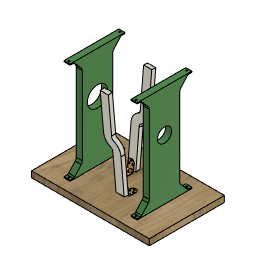
Ventilator_Mk_1_v11 (Autodesk Fusion 360 design; units mm, degrees)
Autodesk Fusion 360 part; units mm, degrees
sketch "Base" plane through (0, 0, 0) normal (0, 0, 1) x (1, 0, 0)
  line L0 (-114.3, 47.625) -> (114.3, 47.625)
  line L1 (114.3, 47.625) -> (114.3, -47.625)
  line L2 (114.3, -47.625) -> (-114.3, -47.625)
  line L3 (-114.3, -47.625) -> (-114.3, 47.625)
  line L4 (-114.3, 47.625) -> (114.3, -47.625) construction
  line L5 (114.3, 47.625) -> (-114.3, -47.625) construction
  line L6 (-95.25, 47.625) -> (-95.25, -47.625)
  line L7 (95.25, 47.625) -> (95.25, -47.625)
  line L8 (-38.1, 47.625) -> (-38.1, -47.625)
  line L9 (38.1, 47.625) -> (38.1, -47.625)
  line L10 (184.15, -117.475) -> (-184.15, -117.475)
  line L11 (-184.15, -117.475) -> (-184.15, 117.475)
  line L12 (-184.15, 117.475) -> (184.15, 117.475)
  line L13 (184.15, 117.475) -> (184.15, -117.475)
  line L14 (38.1323, 0.889) -> (15.9073, 0.889)
  line L15 (19.05, -15.9073) -> (19.05, -38.1323)
  circle A0 centre (22.86, -22.2573) radius 2.54
  circle A1 centre (34.29, -22.2573) radius 2.54
  line L16 (-114.3, -47.625) -> (-114.3, 47.625)
  line L17 (114.3, 47.625) -> (114.3, -47.625)
  line L18 (-114.3, 47.625) -> (-95.25, 47.625)
  line L19 (-95.25, 47.625) -> (-95.25, 85.725)
  line L20 (-95.25, 85.725) -> (-114.3, 85.725)
  line L21 (-114.3, 85.725) -> (-114.3, 47.625)
  line L22 (-114.3, -47.625) -> (-95.25, -47.625)
  line L23 (-95.25, -47.625) -> (-95.25, -85.725)
  line L24 (-95.25, -85.725) -> (-114.3, -85.725)
  line L25 (-114.3, -85.725) -> (-114.3, -47.625)
  line L26 (114.3, 47.625) -> (95.25, 47.625)
  line L27 (95.25, 47.625) -> (95.25, 85.725)
  line L28 (95.25, 85.725) -> (114.3, 85.725)
  line L29 (114.3, 85.725) -> (114.3, 47.625)
  line L30 (114.3, -47.625) -> (95.25, -47.625)
  line L31 (95.25, -47.625) -> (95.25, -85.725)
  line L32 (95.25, -85.725) -> (114.3, -85.725)
  line L33 (114.3, -85.725) -> (114.3, -47.625)
  line L34 (-95.25, -73.025) -> (-114.3, -73.025)
  line L35 (-114.3, 73.025) -> (-95.25, 73.025)
  line L36 (95.25, 73.025) -> (114.3, 73.025)
  line L37 (95.25, -73.025) -> (114.3, -73.025)
  line L38 (-95.25, -73.025) -> (-114.3, -85.725) construction
  line L39 (-114.3, 73.025) -> (-95.25, 85.725) construction
  line L40 (95.25, 73.025) -> (114.3, 85.725) construction
  line L41 (95.25, -85.725) -> (114.3, -73.025) construction
  point P0 (34.29, -22.2573)
  point P1 (22.86, -22.2573)
  point P2 (38.1, -4.445)
  point P3 (-38.1, 4.445)
  point P4 (38.1, -10.795)
  point P5 (-38.1, 10.795)
  point P6 (-104.775, -79.375)
  point P7 (-104.775, 79.375)
  point P8 (104.775, 79.375)
  point P9 (104.775, -79.375)
  dimension "d1" = 95.25
  dimension "d2" = 228.6
  dimension "d3" = 19.05
  dimension "d4" = 19.05
  dimension "d7" = 76.2
  dimension "d8" = 76.2
  dimension "d13" = -69.85
  dimension "d103" = 43.18
  dimension "d104" = 43.18
  dimension "d105" = 6.35
  dimension "d106" = 6.35
  dimension "d216" = 38.1
  dimension "d217" = 38.1
  dimension "d218" = 38.1
  dimension "d219" = 38.1
  dimension "d220" = 12.7
  dimension "d221" = 12.7
  constraint horizontal L0
  constraint perpendicular L0 L1
  constraint parallel L0 L2
  constraint parallel L1 L3
  constraint coincident L4 origin
  constraint coincident L5 origin
  constraint coincident L0 L6.start
  constraint coincident L2 L6.end
  constraint parallel L3 L6
  constraint coincident L0 L7.start
  constraint coincident L2 L7.end
  constraint parallel L6 L7
  constraint coincident L0 L8.start
  constraint coincident L2 L8.end
  constraint perpendicular L2 L8
  constraint coincident L0 L9.start
  constraint coincident L2 L9.end
  constraint perpendicular L2 L9
  constraint coincident L9 P2
  constraint coincident L8 P3
  constraint coincident L9 P4
  constraint coincident L8 P5
  constraint vertical L16
  constraint vertical L17
  constraint horizontal L18
  constraint vertical L19
  constraint horizontal L20
  constraint vertical L21
  constraint collinear L6 L19
  constraint horizontal L22
  constraint vertical L23
  constraint horizontal L24
  constraint vertical L25
  constraint collinear L6 L23
  constraint collinear L2 L22
  constraint horizontal L26
  constraint vertical L27
  constraint horizontal L28
  constraint vertical L29
  constraint collinear L7 L27
  constraint horizontal L30
  constraint vertical L31
  constraint horizontal L32
  constraint vertical L33
  constraint collinear L7 L31
  constraint coincident L23 L34.start
  constraint coincident L25 L34.end
  constraint perpendicular L25 L34
  constraint coincident L19 L35.end
  constraint perpendicular L19 L35
  constraint coincident L27 L36.start
  constraint coincident L29 L36.end
  constraint perpendicular L29 L36
  constraint coincident L31 L37.start
  constraint coincident L33 L37.end
  constraint perpendicular L33 L37
  constraint horizontal L34.end L37.start
  constraint horizontal L35.start L36.start
  constraint midpoint P6 L38
  constraint parallel L40 L41
  constraint midpoint L39 P7
  constraint midpoint L40 P8
  constraint midpoint L41 P9
  measures "d1" distance of L0.end L1.end
  measures "d2" distance of L1 L3
  measures "d3" distance of L3 L6
  measures "d4" distance of L1 L7
  measures "d7" distance of L3 L8
  measures "d8" distance of L1 L9
  measures "d47" distance of P1
  measures "d48" distance of P0
  measures "d49" distance of P0
  measures "d103" distance of L9.end P2
  measures "d104" distance of L8.start P3
  measures "d105" distance of P2 P4
  measures "d106" distance of P3 P5
  measures "d216" distance of L22 L24
  measures "d217" distance of L18 L20
  measures "d218" distance of L26 L28
  measures "d219" distance of L30 L32
  measures "d220" distance of L24 L34
  measures "d221" distance of L20 L35
extrude "Stand Extrude" add sketch "Base" along normal blind 317.5 contours L0 L2 L3 L6 L16 L18 L22 | L0 L1 L2 L7 L17 L26 L30 makes body 1 at (-95.25, 15.875, 105.8333) makes body 2 at (114.3, 15.875, 105.8333)
extrude "StandBaseExtrude" add sketch "Base" along normal blind 31.75 contours L0 L18 L19 L21 L35 | L2 L22 L23 L25 L34 | L0 L26 L27 L29 L36 | L2 L30 L31 L33 L37 bodies 1 2
extrude "StandBaseMountExtrude" add sketch "Base" along normal blind 3.175 contours L19 L20 L21 L35 | L23 L24 L25 L34 | L27 L28 L29 L36 | L31 L32 L33 L37 bodies 1 2
extrude "BaseExtrude" add sketch "Base" against normal blind 19.05 separate body contours L0 L18 L19 L21 L35 | L0 L2 L3 L6 L16 L18 L22 | L0 L2 L6 L8 | L2 L22 L23 L25 L34 | L19 L20 L21 L35 | L0 L2 L8 L9 | L23 L24 L25 L34 | L0 L2 L7 L9 | L0 L26 L27 L29 L36 | L0 L1 L2 L7 L17 L26 L30 | L2 L30 L31 L33 L37 | L27 L28 L29 L36 | L31 L32 L33 L37 | L10 L11 L12 L13 | A0 | A1 makes body 3
hole "Hole5" at (-104.775, -79.375, 0) at (104.775, -79.375, 0) at (104.775, 79.375, 0) at (-104.775, 79.375, 0) direction (0, 0, 1) diameter 5.08 end up to surface (3.175 mm away) bodies 1 2
sketch "L. Stand Cut-Away" plane through (-114.3, 0, 0) normal (-1, 0, 0) x (0, -1, 0)
  line L0 (-73.025, 0) -> (85.725, 0)
  line L1 (85.725, 0) -> (85.725, 3.175)
  line L2 (85.725, 3.175) -> (73.025, 3.175)
  line L3 (73.025, 3.175) -> (73.025, 31.75)
  line L4 (73.025, 31.75) -> (47.625, 31.75)
  line L5 (47.625, 31.75) -> (47.625, 317.5)
  line L6 (47.625, 317.5) -> (-47.625, 317.5)
  line L7 (-47.625, 317.5) -> (-47.625, 31.75)
  line L8 (-47.625, 31.75) -> (-73.025, 31.75)
  line L9 (-73.025, 31.75) -> (-73.025, 3.175)
  line L10 (-73.025, 3.175) -> (-85.725, 3.175)
  line L11 (-85.725, 3.175) -> (-85.725, 0)
  line L12 (-85.725, 0) -> (-73.025, 0)
  line L13 (-47.625, 31.75) -> (-73.025, 3.175)
  line L14 (47.625, 31.75) -> (73.025, 3.175)
  constraint coincident L7.end L8.start
  constraint coincident L9.end L10.start
  constraint coincident L4.end L5.start
  constraint coincident L2.end L3.start
sketch "R. Stand Cut-Away" plane through (95.25, 0, 0) normal (-1, 0, 0) x (0, -1, 0)
  line L0 (-85.725, 0) -> (85.725, 0)
  line L1 (85.725, 0) -> (85.725, 3.175)
  line L2 (85.725, 3.175) -> (73.025, 3.175)
  line L3 (73.025, 3.175) -> (73.025, 31.75)
  line L4 (73.025, 31.75) -> (47.625, 31.75)
  line L5 (47.625, 31.75) -> (47.625, 317.5)
  line L6 (47.625, 317.5) -> (-47.625, 317.5)
  line L7 (-47.625, 317.5) -> (-47.625, 31.75)
  line L8 (-47.625, 31.75) -> (-73.025, 31.75)
  line L9 (-73.025, 31.75) -> (-73.025, 3.175)
  line L10 (-73.025, 3.175) -> (-85.725, 3.175)
  line L11 (-85.725, 3.175) -> (-85.725, 0)
  line L12 (-47.625, 31.75) -> (-73.025, 3.175)
  line L13 (47.625, 31.75) -> (73.025, 3.175)
  constraint coincident L7.end L8.start
  constraint coincident L9.end L10.start
  constraint coincident L4.end L5.start
  constraint coincident L2.end L3.start
extrude "StandBaseAngle" cut sketch "L. Stand Cut-Away" against normal through all contours L3 L4 L14 | L8 L9 L13 bodies 1 2
ref_plane "WorkPlane3" through (0, 0, 158.75) normal (0, 0, 1) x (1, 0, 0)
mirror "Mirror3" about plane through (0, 0, 158.75) normal (0, 0, 1) of "StandBaseExtrude", "StandBaseMountExtrude", "Hole5", "StandBaseAngle"
fillet "Fillet5" radius 12.7 8 edges at (-104.775, -47.625, 31.75) (-104.775, -47.625, 285.75) (-104.775, 47.625, 31.75) (-104.775, 47.625, 285.75) (104.775, -47.625, 31.75) (104.775, -47.625, 285.75) (104.775, 47.625, 31.75) (104.775, 47.625, 285.75) on bodies 1 2
fillet "Fillet6" radius 6.35 8 edges at (-104.775, -73.025, 3.175) (-104.775, 73.025, 3.175) (-104.775, 73.025, 314.325) (-104.775, -73.025, 314.325) (104.775, -73.025, 3.175) (104.775, 73.025, 3.175) (104.775, 73.025, 314.325) (104.775, -73.025, 314.325) on bodies 1 2
sketch "L Stand Holes" plane through (-114.3, 0, 0) normal (-1, 0, 0) x (0, -1, 0)
  line L0 (47.625, 36.5785) -> (47.625, 280.9215)
  line L1 (-47.625, 280.9215) -> (-47.625, 36.5785)
  line L2 (47.625, 0) -> (-47.625, 0)
  line L3 (47.625, 187.325) -> (-47.625, 187.325)
  line L4 (-71.1305, 312.1937) -> (-50.8329, 289.3589)
  line L5 (-50.8329, 28.1411) -> (-71.1305, 5.3063)
  line L6 (-75.8766, 3.175) -> (-85.725, 3.175)
  line L7 (-85.725, 3.175) -> (-85.725, 0)
  line L8 (-85.725, 0) -> (-73.025, 0)
  line L9 (-73.025, 0) -> (85.725, 0)
  line L10 (85.725, 0) -> (85.725, 3.175)
  line L11 (71.1305, 5.3063) -> (50.8329, 28.1411)
  line L12 (50.8329, 289.3589) -> (71.1305, 312.1937)
  line L13 (75.8766, 314.325) -> (85.725, 314.325)
  line L14 (85.725, 314.325) -> (85.725, 317.5)
  line L15 (85.725, 317.5) -> (-73.025, 317.5)
  line L16 (-73.025, 317.5) -> (-85.725, 317.5)
  line L17 (-85.725, 317.5) -> (-85.725, 314.325)
  line L18 (-85.725, 314.325) -> (-75.8766, 314.325)
  arc A0 (-47.625, 280.9215) -> (-50.8329, 289.3589) centre (-60.325, 280.9215) ccw
  arc A1 (-50.8329, 28.1411) -> (-47.625, 36.5785) centre (-60.325, 36.5785) ccw
  arc A2 (-75.8766, 3.175) -> (-71.1305, 5.3063) centre (-75.8766, 9.525) ccw
  line L19 (85.725, 3.175) -> (75.8766, 3.175)
  arc A3 (71.1305, 5.3063) -> (75.8766, 3.175) centre (75.8766, 9.525) ccw
  arc A4 (47.625, 36.5785) -> (50.8329, 28.1411) centre (60.325, 36.5785) ccw
  arc A5 (50.8329, 289.3589) -> (47.625, 280.9215) centre (60.325, 280.9215) ccw
  arc A6 (75.8766, 314.325) -> (71.1305, 312.1937) centre (75.8766, 307.975) ccw
  arc A7 (-71.1305, 312.1937) -> (-75.8766, 314.325) centre (-75.8766, 307.975) ccw
  point P0 (0, 187.325)
  dimension "d232" = 130.175
  constraint coincident L0 L3.start
  constraint coincident L1 L3.end
  constraint perpendicular L1 L3
  constraint midpoint P0 L3
  measures "d232" distance of L3 L15
sketch "R Stand Holes" plane through (95.25, 0, 0) normal (-1, 0, 0) x (0, -1, 0)
  line L0 (47.625, 36.5785) -> (47.625, 280.9215)
  line L1 (-47.625, 280.9215) -> (-47.625, 36.5785)
  line L2 (47.625, 187.325) -> (-47.625, 187.325)
  line L3 (-47.625, 0) -> (47.625, 0)
  line L4 (-71.1305, 312.1937) -> (-50.8329, 289.3589)
  line L5 (-50.8329, 28.1411) -> (-71.1305, 5.3063)
  line L6 (-75.8766, 3.175) -> (-85.725, 3.175)
  line L7 (-85.725, 3.175) -> (-85.725, 0)
  line L8 (-85.725, 0) -> (85.725, 0)
  line L9 (85.725, 0) -> (85.725, 3.175)
  line L10 (71.1305, 5.3063) -> (50.8329, 28.1411)
  line L11 (50.8329, 289.3589) -> (71.1305, 312.1937)
  line L12 (75.8766, 314.325) -> (85.725, 314.325)
  line L13 (85.725, 314.325) -> (85.725, 317.5)
  line L14 (85.725, 317.5) -> (-85.725, 317.5)
  line L15 (-85.725, 317.5) -> (-85.725, 314.325)
  line L16 (-85.725, 314.325) -> (-75.8766, 314.325)
  arc A0 (-47.625, 280.9215) -> (-50.8329, 289.3589) centre (-60.325, 280.9215) ccw
  arc A1 (-50.8329, 28.1411) -> (-47.625, 36.5785) centre (-60.325, 36.5785) ccw
  arc A2 (-75.8766, 3.175) -> (-71.1305, 5.3063) centre (-75.8766, 9.525) ccw
  line L17 (85.725, 3.175) -> (75.8766, 3.175)
  arc A3 (71.1305, 5.3063) -> (75.8766, 3.175) centre (75.8766, 9.525) ccw
  arc A4 (47.625, 36.5785) -> (50.8329, 28.1411) centre (60.325, 36.5785) ccw
  arc A5 (50.8329, 289.3589) -> (47.625, 280.9215) centre (60.325, 280.9215) ccw
  arc A6 (75.8766, 314.325) -> (71.1305, 312.1937) centre (75.8766, 307.975) ccw
  arc A7 (-71.1305, 312.1937) -> (-75.8766, 314.325) centre (-75.8766, 307.975) ccw
  point P0 (0, 187.325)
  dimension "d233" = 130.175
  constraint coincident L0 L2.start
  constraint coincident L1 L2.end
  constraint perpendicular L1 L2
  constraint midpoint L2 P0
  measures "d233" distance of L2 L14
hole "Hole1" at (-114.3, 0, 187.325) direction (1, 0, 0) diameter 63.5 end up to surface (19.05 mm away) bodies 1
hole "Hole3" at (95.25, 0, 187.325) direction (1, 0, 0) diameter 44.45 end through all bodies 2
sketch "L. Stand Base" plane through (0, 0, 0) normal (0, 0, -1) x (1, 0, 0)
  line L0 (-146.05, -47.625) -> (-63.5, -47.625)
  line L1 (-63.5, -47.625) -> (-63.5, 47.625)
  line L2 (-63.5, 47.625) -> (-146.05, 47.625)
  line L3 (-146.05, 47.625) -> (-146.05, -47.625)
  line L4 (-133.35, -47.625) -> (-133.35, 47.625)
  line L5 (-76.2, -47.625) -> (-76.2, 47.625)
  line L6 (-133.35, 0) -> (-146.05, 0)
  line L7 (-63.5, 0) -> (-76.2, 0)
  circle A0 centre (-104.775, 79.375) radius 2.54
  circle A1 centre (-104.775, -79.375) radius 2.54
  line L8 (-114.3, 85.725) -> (-114.3, -73.025)
  line L9 (-114.3, -73.025) -> (-114.3, -85.725)
  line L10 (-114.3, -85.725) -> (-95.25, -85.725)
  line L11 (-95.25, -85.725) -> (-95.25, 85.725)
  line L12 (-95.25, 85.725) -> (-114.3, 85.725)
  point P0 (-139.7, 0)
  point P1 (-139.7, 34.925)
  point P2 (-139.7, -34.925)
  point P3 (-69.85, -34.925)
  point P4 (-69.85, 0)
  point P5 (-69.85, 34.925)
  dimension "d177" = 12.7
  dimension "d178" = 12.7
  dimension "d180" = 95.25
  dimension "d183" = 12.7
  dimension "d184" = 12.7
  constraint horizontal L0
  constraint vertical L1
  constraint horizontal L2
  constraint vertical L3
  constraint coincident L0 L4.start
  constraint coincident L2 L4.end
  constraint perpendicular L2 L4
  constraint coincident L0 L5.start
  constraint coincident L2 L5.end
  constraint perpendicular L2 L5
  constraint vertical P0 P1
  constraint vertical P1 P2
  constraint midpoint L4 L6.start
  constraint midpoint L3 L6.end
  constraint midpoint P0 L6
  constraint vertical P4 P5
  constraint vertical P3 P5
  constraint horizontal P1 P5
  constraint horizontal P0 P4
  constraint horizontal P2 P3
  constraint midpoint L1 L7.start
  constraint midpoint L5 L7.end
  constraint midpoint P4 L7
  measures "d177" distance of L3 L4
  measures "d178" distance of L1 L5
  measures "d180" distance of L0 L2
  measures "d183" distance of L2 P1
  measures "d184" distance of L0 P2
sketch "Arm Path" plane through (0, 0, 0) normal (0, 1, 0) x (1, 0, 0)
  line L0 (0, 0) -> (0, -116.84)
  line L1 (-25.4, -162.56) -> (-25.4, -279.4)
  line L2 (0, -116.84) -> (-25.4, -162.56) construction
  line L3 (-25.4, -139.7) -> (0, -139.7) construction
  line L4 (0, -116.84) -> (0, -139.7)
  line L5 (0, -139.7) -> (-12.7, -139.7)
  line L6 (-12.7, -139.7) -> (-25.4, -139.7)
  line L7 (-25.4, -139.7) -> (-25.4, -162.56)
  spline S0 degree 4 poles (0, -116.84) (0, -139.7) (-12.7, -139.7) (-25.4, -139.7) (-25.4, -162.56) knots 0 0 0 0 0 1 1 1 1 1
  point P0 (-12.7, -139.7)
  dimension "d20" = 25.4
  dimension "d22" = 25.4
  dimension "d33" = 279.4
  dimension "d168" = 139.7
  constraint coincident L0.start origin
  constraint vertical L0
  constraint parallel L0 L1
  constraint midpoint L2 P0
  constraint horizontal L3
  constraint vertical L0.start L3.end
  constraint midpoint P0 L3
  constraint coincident L3.end L4.end
  constraint coincident P0 L5.end
  constraint coincident L3.start L6.end
  measures "d20" distance of L0 L1
  measures "d22" distance of L3.start L3.end
  measures "d33" vertical distance of L0.start L1.end
  measures "d168" vertical distance of L0.start P0
sketch "Arm Base" plane through (0, 0, 0) normal (0, 0, 1) x (1, 0, 0)
  line L0 (12.7, 6.35) -> (-12.7, 6.35)
  line L1 (-12.7, 6.35) -> (-12.7, -6.35)
  line L2 (-12.7, -6.35) -> (12.7, -6.35)
  line L3 (12.7, -6.35) -> (12.7, 6.35)
  line L4 (12.7, 6.35) -> (-12.7, -6.35) construction
  line L5 (-12.7, 6.35) -> (12.7, -6.35) construction
  dimension "d25" = 25.4
  dimension "d26" = 12.7
  constraint horizontal L0
  constraint perpendicular L0 L1
  constraint parallel L0 L2
  constraint parallel L1 L3
  constraint coincident L4 origin
  constraint coincident L5 origin
  measures "d25" distance of L1.end L2.end
  measures "d26" distance of L0.end L1.end
sweep "Sweep1" add profiles "Arm Base" path "Arm Path" along L0 S0 L1 section 1 separate body makes body 4
sketch "Arm Angle" plane through (-12.7, 0, 0) normal (-1, 0, 0) x (0, -1, 0)
  line L0 (-6.35, 0) -> (6.35, 0)
  line L1 (6.35, 0) -> (6.35, 116.84)
  line L2 (6.35, 116.84) -> (-6.35, 116.84)
  line L3 (-6.35, 116.84) -> (-6.35, 0)
  line L4 (-6.35, 0) -> (6.35, 3.403)
  dimension "d35" = 15
  constraint coincident L0.start L3.end
  constraint coincident L1 L4.end
  measures "d35" angle of L0 L4
extrude "Extrude3" cut sketch "Arm Angle" against normal through all contours L0 L1 L4 bodies 4
move_body "Move1" bodies 4 to x (1, 0, 0) y (0, 1, 0) z (0, 0, 1) at (0, -76.2, 0)
copy_body "CopyPasteBodies2" bodies 4 makes body 5
move_body "Move3" bodies 5 to x (-1, 0, 0) y (0, -1, 0) z (0, 0, 1) at (-25.4101, -25.4102, 0)
sketch "Hinge Base" plane through (0, 0, 0) normal (0, 0, 1) x (1, 0, 0)
  line L0 (-38.1, 41.3073) -> (-38.1, 15.9073)
  line L1 (-33.3375, 9.5573) -> (-38.1, 15.9073)
  line L2 (-33.3375, 9.5573) -> (-23.8125, 9.5573)
  line L3 (-38.1, 41.3073) -> (-19.05, 41.3073)
  line L4 (-23.8125, 9.5573) -> (-19.05, 15.9073)
  line L5 (-19.05, 15.9073) -> (-19.05, 41.3073)
  line L6 (-114.3, 47.625) -> (114.3, 47.625)
  point P0 (-38.1, -47.625)
  point P1 (-33.3375, 9.5573)
  dimension "d38" = 25.4
  dimension "d39" = 4.7625
  dimension "d40" = 6.35
  dimension "d41" = 9.525
  dimension "d42" = 19.05
  dimension "d43" = 6.3177
  constraint vertical L0
  constraint vertical L0.end P0
  constraint coincident P1 L1.start
  constraint perpendicular L0 L2
  constraint perpendicular L0 L3
  constraint horizontal L0.end L4.end
  constraint vertical L3.end L4.end
  measures "d38" distance of L0.start L0.end
  measures "d39" horizontal distance of L0.end P1
  measures "d40" vertical distance of L0.end P1
  measures "d41" distance of P1 L2.end
  measures "d42" distance of L0.start L3.end
  measures "d43" distance of L3 L6
extrude "Extrude4" add sketch "Hinge Base" along normal blind 0.889 separate body makes body 6
sketch "Hinge Holes" plane through (0, 0, 0.889) normal (0, 0, 1) x (-1, 0, 0)
  line L0 (33.3375, -9.5573) -> (23.8125, -9.5573)
  line L1 (23.8125, -9.5573) -> (19.05, -15.9073)
  line L2 (19.05, -15.9073) -> (19.05, -41.3073)
  line L3 (19.05, -41.3073) -> (38.1, -41.3073)
  line L4 (38.1, -41.3073) -> (38.1, -15.9073)
  line L5 (38.1, -15.9073) -> (33.3375, -9.5573)
  point P0 (28.3981, -13.3673)
  point P1 (34.29, -22.2573)
  point P2 (22.86, -22.2573)
  dimension "d46" = 3.81
  dimension "d47" = 3.81
  dimension "d48" = 3.81
  dimension "d49" = 12.7
  constraint horizontal P1 P2
  measures "d46" distance of L0 P0
  measures "d47" distance of L2 P2
  measures "d48" distance of L4 P1
  measures "d49" distance of L0 P1
hole "Hole2" at (-22.86, 22.2573, 0.889) at (-34.29, 22.2573, 0.889) at (-28.3981, 13.3673, 0.889) direction (0, 0, -1) diameter 5.08 end through all bodies 6
sketch "Hinge LJ Joint" plane through (-19.05, 0, 0) normal (1, 0, 0) x (0, 1, 0)
  line L0 (15.9073, 0) -> (41.3073, 0)
  line L1 (41.3073, 0) -> (41.3073, 0.889)
  line L2 (41.3073, 0.889) -> (15.9073, 0.889)
  line L3 (15.9073, 0.889) -> (15.9073, 0)
  line L4 (41.3073, 0.889) -> (41.3073, 4.064)
  circle A0 centre (38.1323, 4.064) radius 3.175
  circle A1 centre (38.1323, 4.064) radius 2.0581
  arc A2 (37.2433, 0) -> (41.3073, 4.064) centre (37.2433, 4.064) ccw
  dimension "d54" = 3.175
  dimension "d57" = -1.1169
  constraint coincident L1.end L2.start
  constraint perpendicular L2 L4
  constraint tangent L4 A0
  constraint tangent L2 A0
  constraint coincident L4.end A0
  constraint tangent L0 A2
  constraint tangent L4 A2
  constraint coincident L0 A2.start
  measures "d54" radius of A0
extrude "Extrude5" add sketch "Hinge LJ Joint" against normal blind 9.525 contours L2 A0 A2 | A0 | A1 bodies 6
extrude "Extrude6" cut sketch "Hinge LJ Joint" against normal through all contours L0 L1 L2 A2 | L2 L4 A2 | A1 bodies 6
sketch "Sketch13" plane through (0, 0, 0.889) normal (0, 0, 1) x (-1, 0, 0)
  line L0 (28.575, -39.7801) -> (38.1, -39.7801)
  line L1 (38.1, -39.7801) -> (38.1, -15.9073)
  line L2 (38.1, -15.9073) -> (33.3375, -9.5573)
  line L3 (33.3375, -9.5573) -> (23.8125, -9.5573)
  line L4 (23.8125, -9.5573) -> (19.05, -15.9073)
  line L5 (19.05, -15.9073) -> (19.05, -38.1323)
  line L6 (19.05, -38.1323) -> (28.575, -38.1323)
  line L7 (28.575, -38.1323) -> (28.575, -39.7801)
  circle A0 centre (28.3981, -13.3673) radius 2.54
  circle A1 centre (22.86, -22.2573) radius 2.54
  circle A2 centre (34.29, -22.2573) radius 2.54
  line L8 (38.1, -39.7801) -> (28.5846, -39.7801)
  line L9 (28.5846, -39.7801) -> (28.5846, -34.9541)
  line L10 (28.5846, -34.9541) -> (38.1, -34.9541)
  line L11 (38.1, -34.9541) -> (38.1, -39.7801)
  dimension "d76" = 4.826
  constraint horizontal L8
  constraint vertical L9
  constraint horizontal L10
  constraint vertical L11
  constraint coincident L0.end L1.start
  measures "d76" distance of L0.end L10.end
extrude "Extrude8" cut sketch "Sketch13" against normal through all contours L0 L1 L8 L9 L10 L11 bodies 6
copy_body "CopyPasteBodies1" bodies 6 makes body 7
move_body "Move2" bodies 7 to x (1, 0, 0) y (0, 1, 0) z (0, 0, 1) at (38.1, 0, 0)
sketch "Hinge UJ Joint" plane through (19.05, 0, 0) normal (1, 0, 0) x (0, 1, 0)
  circle A0 centre (38.1323, 4.064) radius 2.0581
  circle A1 centre (38.1323, 4.064) radius 2.0581
  arc A2 (37.2433, 0) -> (41.3073, 4.064) centre (37.2433, 4.064) ccw
  arc A3 (41.3073, 4.064) -> (38.1323, 0.889) centre (38.1323, 4.064) ccw
  line L0 (38.1323, 0.889) -> (15.9073, 0.889)
  line L1 (15.9073, 0.889) -> (15.9073, 0)
  line L2 (15.9073, 0) -> (37.2433, 0)
  constraint concentric A0 A1
extrude "Extrude7" add sketch "Hinge UJ Joint" against normal blind 19.05 contours A0 A1 bodies 7
copy_body "Body->Comp1" bodies 7 removing the originals makes body 8 in component "Hinge UJ"
copy_body "Body->Comp2" bodies 6 removing the originals makes body 9 in component "Hinge LJ"
copy_body "Body->Comp3" bodies 5 removing the originals makes body 10 in component "Back Arm "
copy_body "Body->Comp4" bodies 3 removing the originals makes body 11 in component "Base"
copy_body "Body->Comp5" bodies 1 removing the originals makes body 12 in component "L. Stand"
copy_body "Body->Comp6" bodies 2 removing the originals makes body 13 in component "R. Stand"
copy_body "Body->Comp7" bodies 4 removing the originals makes body 14 in component "Front Arm"
component "Hinge UJ" placed x (-1, 0, 0) y (0, -0.087156, -0.996195) z (0, -0.996195, 0.087156) at (-19.05, 40.392, 41.697)
component "Hinge LJ" placed x (1, 0, 0) y (0, 1, 0) z (0, 0, 1) at (0, -5.1123, 0)
component "Back Arm " placed x (1, 0, 0) y (0, 0.996195, -0.087156) z (0, 0.087156, 0.996195) at (0.0101, -7.1246, 8.4686)
component "Hinge UJ" placed x (1, 0, 0) y (0, 0.087156, -0.996195) z (0, 0.996195, 0.087156) at (19.05, -40.392, 41.697)
component "Hinge LJ" placed x (-1, 0, 0) y (0, -1, 0) z (0, 0, 1) at (0, 5.1123, 0)
component "Base" placed x (1, 0, 0) y (0, 1, 0) z (0, 0, 1) at (0, 0, 0)
component "L. Stand" placed x (1, 0, 0) y (0, 1, 0) z (0, 0, 1) at (0, 0, 0)
component "R. Stand" placed x (1, 0, 0) y (0, 1, 0) z (0, 0, 1) at (0, 0, 0)
component "Front Arm" placed x (1, 0, 0) y (0, 0.996195, 0.087156) z (0, -0.087156, 0.996195) at (25.4, 32.4382, 10.6832)
equation "d1 = 3 3/4\""
equation "d4 = d3"
equation "d8 = d7"
equation "d9 = 12.5 in"
equation "d39 = ( 3 / 16 ) * 1 in"
equation "d41 = ( 6 / 16 ) * 1 in"
equation "d168 = d33 / 2"
equation "d178 = d177"
equation "d184 = d183"
equation "d209 = d9 / 2"
equation "d217 = d216"
equation "d218 = d216"
equation "d219 = d216"
equation "d221 = d220"
equation "d233 = d232"
named bodies: "L. Stand", "R. Stand", "Base", "Front Arm", "Hinge LJ", "Hinge UJ", "Back Arm"
